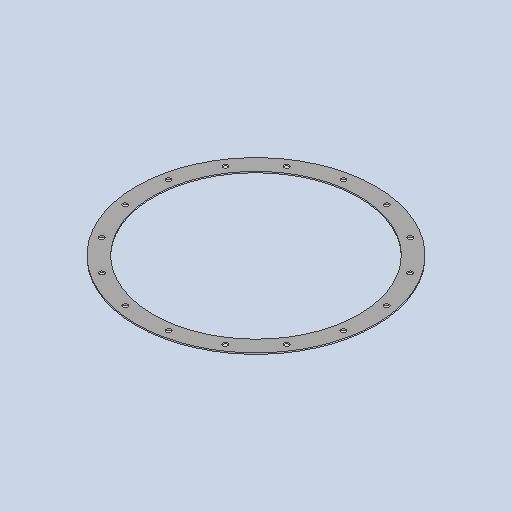
# Autodesk Inventor part: ДМФ 041 кольцо под шпильки КОРМА
Saved by Autodesk Inventor 2025 (Build 290162010, 162A)
## iProperties
Created: 2024-04-23
Part Number: ДМФ 041 кольцо под шпильки КОРМА
Material: Generic
Document SubType Name: Sheet Metal
Designer: admin
Density: 1 g/cm^3
Appearance: Default
Sheet Metal Rule: Default
Flat Pattern Width: 57 cm
Flat Pattern Length: 57 cm
Flat Pattern Area: 3249 cm^2
Sheet Metal Width: 570,000 mm
Sheet Metal Length: 570,000 mm
Sheet Metal Area: 324900,000 mm^2
Stock Number: ДМФ 041 кольцо под шпильки КОРМА
Author: admin
Autodesk Inventor part; units mm, degrees
ref_plane "YZ Plane" through (0, 0, 0) normal (1, 0, 0) x (0, 1, 0)
ref_plane "XZ Plane" through (0, 0, 0) normal (0, 1, 0) x (-1, 0, 0)
ref_plane "XY Plane" through (0, 0, 0) normal (0, 0, 1) x (1, 0, 0)
sketch "Sketch1" plane through (0, 0, 0) normal (0, 0, 1) x (1, 0, 0)
  circle A0 centre (0, 0) radius 245
  circle A1 centre (0, 0) radius 285
  circle A2 centre (0, 0) radius 265 construction
  line L0 (0, 285) -> (0, 245) construction
  point P0 (0, 265)
  dimension "d9" = 530
  dimension "d11" = 40
extrude "Plate1" add sketch "Sketch1" along normal blind 3
sketch "Sketch2" plane through (0, 0, 3) normal (0, 0, 1) x (1, 0, 0)
  circle A0 centre (0, 0) radius 245 construction
  circle A1 centre (0, 0) radius 285 construction
  circle A2 centre (0, 0) radius 285 projected
  circle A3 centre (0, 0) radius 245 projected
  line L0 (0, 0) -> (0, -285) construction
  line L1 (0, 0) -> (-55.6007, -279.5238) construction
  line L2 (-47.7971, -240.2924) -> (-55.6007, -279.5238) construction
  circle A4 centre (-51.6989, -259.9081) radius 6
  dimension "d20" = 11.25
  dimension "d21" = 12
  constraints: 6 end point, 2 point on circle, 1 centre point, 1 collinear, 1 midpoint, 1 point on line, 1 vertical, 2 other
  measures "d20" angle of L0 L1
  measures "d21" diameter of A4
extrude "Extrusion1" cut sketch "Sketch2" against normal through all contours A4
sketch "Sketch3" plane through (0, 0, 3) normal (0, 0, 1) x (1, 0, 0)
  circle A0 centre (0, 0) radius 245 projected
  line L0 (-245, 0) -> (-250, 0) construction
  line L1 (-250, 5) -> (-250, -5)
  line L2 (-250, 5) -> (-244.949, 5)
  line L3 (-250, -5) -> (-244.949, -5)
  line L4 (245, 0) -> (250, 0) construction
  line L5 (250, 5) -> (250, -5)
  line L6 (250, 5) -> (244.949, 5)
  line L7 (250, -5) -> (244.949, -5)
  dimension "d23" = 5
  dimension "d24" = 10
  constraints: 16 end point, 6 horizontal, 6 point on circle, 2 equal length, 2 horizontal alignment, 2 midpoint, 2 vertical
  measures "d23" distance of L0.end L0.start
  measures "d24" distance of L1.start L1.end
extrude "Extrusion2" [suppressed]
pattern_circular "Circular Pattern2" count 16 over 360 about axis through (0, 0, 0) along (0, 0, 1) of "Extrusion1"
equation "\"d9\" = Шпил_пласт_КОРМА_диам_центров"
equation "\"d11\" = Шпил_пласт_КОРМА_ширина"
equation "\"d21\" = Шпил_пласт_КОРМА_диам_шпильки"
equation "\"d2\" = Thickness"
equation "\"BendRadius\" = Thickness"
equation "\"BendReliefWidth\" = Thickness"
equation "\"BendReliefDepth\" = 0.5 * Thickness"
equation "\"CornerReliefSize\" = 4 * Thickness"
equation "\"MinimumRemnant\" = 2 * Thickness"
equation "\"TransitionRadius\" = BendRadius"
equation "\"JacobiRadiusSize\" = BendRadius"
equation "\"GapSize\" = Thickness"
equation "\"Шпил_пласт_КОРМА_диам_центров\" = 530"
equation "\"Шпил_пласт_КОРМА_ширина\" = 40"
equation "\"Шпил_пласт_КОРМА_диам_шпильки\" = 12"
equation "\"Thickness\" = 3"
body "Solid1"
